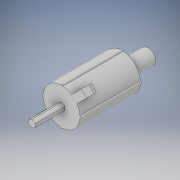
# Autodesk Inventor part: eix bobina
Saved by Autodesk Inventor 2019 (Build 230136000, 136)
## iProperties
Created: 2018-08-16
Part Number: eix bobina
Material: Genérico
Document SubType Name: Modeling
Designer: Albert Garangou Culebras
Density: 1 g/cm^3
Appearance: Valor por defecto
Author: Albert Garangou Culebras
Autodesk Inventor part; units mm, degrees
ref_plane "YZ Plane" through (0, 0, 0) normal (1, 0, 0) x (0, 1, 0)
ref_plane "XZ Plane" through (0, 0, 0) normal (0, 1, 0) x (-1, 0, 0)
ref_plane "XY Plane" through (0, 0, 0) normal (0, 0, 1) x (1, 0, 0)
sketch "Boceto1" plane through (0, 0, 0) normal (0, 0, 1) x (1, 0, 0)
  circle A0 centre (0, 0) radius 24.5
  line L0 (0, 24.5) -> (0, 26)
  arc A1 (1.4693, 24.4559) -> (0, 25.97) centre (0, 24.5) ccw
  arc A2 (0, 25.97) -> (-1.4693, 24.4559) centre (0, 24.5) ccw
  line L1 (0, -24.5) -> (0, -26)
  arc A3 (0, -26) -> (1.4993, -24.4541) centre (0, -24.5) ccw
  arc A4 (-1.4993, -24.4541) -> (0, -26) centre (0, -24.5) ccw
  line L2 (24.5, 0) -> (25.97, 0)
  line L3 (-24.5, 0) -> (-26, 0)
  arc A5 (-24.4541, 1.4993) -> (-24.4541, -1.4993) centre (-24.5, 0) ccw
  arc A6 (24.4559, -1.4693) -> (24.4559, 1.4693) centre (24.5, 0) ccw
  dimension "d0" = 49
  dimension "d1" = 1.5
  dimension "d2" = 1.5
  dimension "d4" = 1.5
  constraints: 14 point on circle, 8 end point, 6 centre point, 6 coincident, 2 horizontal, 2 vertical, 15 other
  measures "d1" distance of L0.start L0.end
  measures "d2" distance of L1.start L1.end
  measures "d4" distance of L3.start L3.end
extrude "Extrusión1" add sketch "Boceto1" along normal blind 81
sketch "Boceto2" plane through (0, 0, 81) normal (0, 0, 1) x (1, 0, 0)
  line L0 (0, 5) -> (4.3301, 2.5)
  line L1 (4.3301, 2.5) -> (4.3301, -2.5)
  line L2 (4.3301, -2.5) -> (0, -5)
  line L3 (0, -5) -> (-4.3301, -2.5)
  line L4 (-4.3301, -2.5) -> (-4.3301, 2.5)
  line L5 (-4.3301, 2.5) -> (0, 5)
  point P0 (0, 0)
  point P1 (0, 0)
  constraints: 12 end point, 1 coincident, 13 other
extrude "Extrusión2" add sketch "Boceto2" along normal blind 40
sketch "Boceto3" plane through (0, 0, 81) normal (0, 0, 1) x (1, 0, 0)
  arc A0 (24.4559, 1.4693) -> (1.4693, 24.4559) centre (0, 0) ccw projected
  arc A1 (24.4559, 1.4693) -> (1.4693, 24.4559) centre (0, 0) ccw
  line L0 (17.3241, 17.3241) -> (0, 0)
  line L1 (17.3241, 17.3241) -> (13.4463, 20.4804)
  line L2 (17.3241, 17.3241) -> (20.4804, 13.4463)
  line L3 (20.4804, 13.4463) -> (27.5868, 20.4819)
  line L4 (13.4463, 20.4804) -> (20.4819, 27.5868)
  line L5 (20.4819, 27.5868) -> (27.5868, 20.4819)
  dimension "d9" = 5
  dimension "d10" = 5
  dimension "d12" = 10
  dimension "d13" = 10
  constraints: 12 end point, 7 point on circle, 1 centre point, 1 coincident
  measures "d9" distance of L0.start L1.end
  measures "d10" distance of L2.start L2.end
  measures "d12" distance of L2.end L3.end
  measures "d13" distance of L1.end L4.end
extrude "Extrusión3" add sketch "Boceto3" against normal blind 10 contours A0 L4 L5 L3
sketch "Boceto4" plane through (27.5868, 20.4819, 71) normal (0.7071068, 0.7071068, 0) x (-0.7071068, 0.7071068, 0)
  line L0 (9.9978, 0) -> (10.0478, 0) projected
  line L1 (0.05, 10) -> (-11.2301, 10) projected
  line L2 (10.0478, 0) -> (0.05, 0)
  line L3 (0.05, 0) -> (0.05, 10)
  line L4 (0.05, 10) -> (10.0478, 10)
  line L5 (10.0478, 10) -> (10.0478, 0)
  point P0 (5.0239, -71)
  constraints: 8 end point, 2 parallel, 1 horizontal, 1 perpendicular
extrude "Extrusión4" add sketch "Boceto4" along normal blind 10
sketch "Boceto5" plane through (0, 0, 71) normal (0, 0, -1) x (-1, 0, 0)
  line L0 (-34.6225, 27.5883) -> (-27.553, 34.6578) projected
  line L1 (-27.6046, 34.6062) -> (-34.6225, 27.5883)
  line L2 (-34.6225, 27.5883) -> (-27.5868, 20.482)
  line L3 (-20.4819, 27.5868) -> (-27.553, 34.6578) projected
  line L4 (-27.553, 34.6578) -> (-20.4819, 27.5868)
  line L5 (-20.4804, 13.4463) -> (-27.5868, 20.4819) projected
  line L6 (-20.4819, 27.5868) -> (-27.5868, 20.4819)
  line L7 (-20.4819, 27.5868) -> (-13.4463, 20.4804) projected
  line L8 (-20.4819, 27.5868) -> (-27.553, 34.6578)
  line L9 (-27.553, 34.6578) -> (-34.6225, 27.5883)
  line L10 (-27.5514, 20.5172) -> (-34.6225, 27.5883) projected
  line L11 (-27.5868, 20.4819) -> (-34.6225, 27.5883)
  line L12 (-27.5514, 20.5172) -> (-20.4819, 27.5868)
  point P0 (0, 0)
  dimension "d18" = 10
  dimension "d19" = 10
  constraints: 16 end point, 4 collinear, 2 point on line, 1 perpendicular
  measures "d18" distance of L0.start L2.end
  measures "d19" distance of L0.end L3.start
extrude "Extrusión5" add sketch "Boceto5" along normal blind 10 contours L0 L3 L6 L10
sketch "Boceto6" plane through (27.5514, 20.5172, 81) normal (0.7071068, -0.7071068, 0) x (-0.7071068, -0.7071068, 0)
  line L0 (0, 10) -> (0, 20) projected
  line L1 (-10, 10) -> (0, 20)
  line L2 (-10, 20) -> (0, 20) projected
  line L3 (-10, 10) -> (-10, 20)
  line L4 (-10, 20) -> (0, 20)
  point P0 (33.9897, 81)
  constraints: 6 end point, 1 collinear, 1 vertical
extrude "Extrusión6" cut sketch "Boceto6" against normal blind 13.25
sketch "Boceto7" plane through (0, 0, 81) normal (0, 0, 1) x (1, 0, 0)
  arc A0 (-24.4559, -1.4693) -> (-1.6038, -24.4475) centre (0, 0) ccw
  line L0 (0, 0) -> (-17.3717, -17.2764)
  arc A1 (-24.4541, -1.4993) -> (-1.4993, -24.4541) centre (0, 0) ccw projected
  line L1 (-17.3717, -17.2764) -> (-13.5025, -20.4434)
  line L2 (-17.3717, -17.2764) -> (-20.5173, -13.3899)
  arc A2 (20.4804, 13.4463) -> (13.4463, 20.4804) centre (0, 0) ccw projected
  line L3 (13.4463, 20.4804) -> (-20.5173, -13.3899)
  arc A3 (24.4559, 1.4693) -> (20.4804, 13.4463) centre (0, 0) ccw projected
  line L4 (20.4804, 13.4463) -> (-13.5025, -20.4434)
  line L5 (-26.5537, -33.3169) -> (-33.5475, -26.2068)
  line L6 (-26.5537, -33.3169) -> (-13.5025, -20.4434)
  line L7 (-33.5475, -26.2068) -> (-20.5173, -13.3899)
  dimension "d24" = 5
  dimension "d25" = 5
  constraints: 16 end point, 6 point on circle, 1 centre point, 1 coincident, 1 perpendicular
  measures "d24" distance of L0.end L1.end
  measures "d25" distance of L0.end L2.end
extrude "Extrusión7" add sketch "Boceto7" against normal blind 10 contours A0 L6 L5 L7
sketch "Boceto10" plane through (0, 0, 0) normal (0, 0, -1) x (-1, 0, 0)
  circle A0 centre (0, 0) radius 7.5
  dimension "d37" = 15
  constraints: 1 centre point, 1 coincident
  measures "d37" diameter of A0
extrude "Extrusión9" add sketch "Boceto10" along normal blind 35
sketch "Boceto12" plane through (0, 0, 0) normal (0, 0, -1) x (-1, 0, 0)
  circle A0 centre (0, 0) radius 10
  dimension "d40" = 20
  constraints: 1 centre point, 1 coincident
  measures "d40" diameter of A0
extrude "Extrusión10" add sketch "Boceto12" along normal blind 35
sketch "Boceto15" plane through (-26.5537, -33.3169, 71) normal (0.7022437, -0.7119367, 0) x (0.7119367, 0.7022437, 0)
  line L0 (0.0139, 0) -> (18.2912, 0) projected
  line L1 (0.0139, 0) -> (5.0139, 0)
  line L2 (0.0139, 0) -> (5.0139, -5)
  line L3 (0.0139, 0) -> (7.085, 0) construction
  line L4 (5.0139, 0) -> (10.0139, 0)
  line L5 (5.0139, -5) -> (10.0139, -10)
  line L6 (10.0139, -10) -> (10.0139, 0)
  point P0 (42.3012, -71)
  dimension "d47" = 45
  dimension "d50" = 5
  constraints: 12 end point, 2 point on line, 1 equal length, 1 horizontal, 1 vertical
  measures "d47" angle of L2 L3
  measures "d50" distance of L1.end L4.end
extrude "Extrusión12" add sketch "Boceto15" against normal blind 10
sketch "Boceto16" plane through (20.4804, 13.4463, 71) normal (0.7035624, -0.7106335, 0) x (0.7106335, 0.7035624, 0)
  line L0 (18.3333, 10) -> (18.3333, 0)
  line L1 (18.3333, 10) -> (19.9996, 10)
  line L2 (19.9996, 10) -> (19.9996, 0) projected
  line L3 (19.9996, 10) -> (19.9996, 0)
  line L4 (19.9996, 0) -> (18.3333, 0)
  line L5 (18.3333, 0) -> (19.9996, 0)
  point P0 (-24.0144, -71)
  point P1 (-0.0497, 0)
  constraints: 10 end point, 1 collinear, 1 horizontal, 1 perpendicular, 1 vertical
extrude "Extrusión13" cut sketch "Boceto16" against normal blind 72.5
sketch "Boceto17" plane through (27.5514, 20.5172, 81) normal (0.7071068, -0.7071068, 0) x (-0.7071068, -0.7071068, 0)
  line L0 (-8.3337, 10) -> (-8.3337, 0) projected
  line L1 (-8.3337, 10) -> (0, 10)
  line L2 (0, 10) -> (0, 20) projected
  line L3 (0, 10) -> (0, 20)
  line L4 (0, 20) -> (-10, 10)
  line L5 (-10, 10) -> (-8.3337, 10)
  point P0 (33.9897, 81)
  constraints: 8 end point, 2 collinear, 1 horizontal, 1 point on line
extrude "Extrusión14" cut sketch "Boceto17" against normal blind 90
sketch "Boceto18" plane through (27.5514, 20.5172, 81) normal (0.7071068, -0.7071068, 0) x (-0.7071068, -0.7071068, 0)
  line L0 (0, 10) -> (-8.3337, 10) projected
  line L1 (-8.3337, 10) -> (1.6663, 10)
  line L2 (1.6663, 10) -> (1.6663, 20)
  line L3 (-8.3337, 10) -> (1.6663, 20)
  point P0 (33.9897, 81)
  dimension "d56" = 10
  dimension "d57" = 10
  constraints: 6 end point, 1 collinear, 1 perpendicular
  measures "d56" distance of L0.end L1.end
  measures "d57" distance of L1.end L2.end
extrude "Extrusión15" add sketch "Boceto18" against normal blind 10
